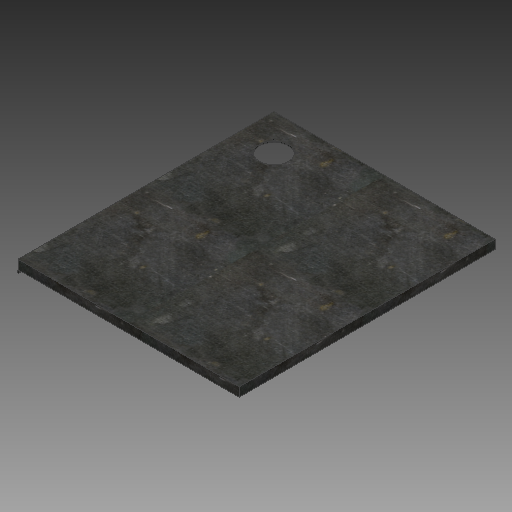
# Autodesk Inventor part: lid
Saved by Autodesk Inventor 2018 (Build 220112000, 112)
## iProperties
Created: 2018-08-03
Part Number: lid
Material: Steel
Document SubType Name: Modeling
Designer: Cole Tucker
Density: 7.85 g/cm^3
Appearance: Plate
Mass: 1610.8 g
Surface Area: 2598 cm^2
Volume: 205.197 cm^3
Author: Cole Tucker
Autodesk Inventor part; units mm, degrees
ref_plane "YZ Plane" through (0, 0, 0) normal (1, 0, 0) x (0, 1, 0)
ref_plane "XZ Plane" through (0, 0, 0) normal (0, 1, 0) x (-1, 0, 0)
ref_plane "XY Plane" through (0, 0, 0) normal (0, 0, 1) x (1, 0, 0)
sketch "Sketch1" plane through (0, 0, 0) normal (0, 1, 0) x (-1, 0, 0)
  line L0 (0, 0) -> (361.95, 0)
  line L1 (361.95, 0) -> (361.95, -312.7502)
  line L2 (361.95, -312.7502) -> (0, -312.7502)
  line L3 (0, -312.7502) -> (0, 0)
  dimension "d0" = 361.95
  dimension "d1" = 312.7502
  constraints: 8 end point, 2 parallel, 1 horizontal, 1 perpendicular
  measures "d0" distance of L1.end L2.end
  measures "d1" distance of L0.end L1.end
extrude "Extrusion1" add sketch "Sketch1" along normal blind 12.7
shell "Shell1" thickness 1.5875 removed faces 1 at (-120.65, 0, -104.2501)
sketch "Sketch2" plane through (0, 0, 0) normal (1, 0, 0) x (0, 0, -1)
  line L0 (0, 0) -> (0, -3.175)
  arc A0 (0, -1.5875) -> (1.5875, -3.175) centre (0, -3.175) ccw
  line L1 (1.5875, -3.175) -> (1.5875, 0)
  line L2 (312.7502, 0) -> (0, 0) projected
  line L3 (1.5875, 0) -> (0, 0)
  dimension "d5" = 3.175
  dimension "d6" = 3.175
  constraints: 6 end point, 2 point on circle, 2 vertical, 1 centre point, 1 coincident, 1 midpoint, 1 perpendicular, 1 tangent
  measures "d5" distance of L0.start L0.end
  measures "d6" diameter of A0
extrude "Extrusion2" add sketch "Sketch2" against normal up to surface (361.95 mm away)
sketch "Sketch3" plane through (0, 12.7, 0) normal (0, 1, 0) x (1, 0, 0)
  line L0 (-361.95, 312.7502) -> (-361.95, 0) construction
  line L1 (-361.95, 0) -> (-311.15, 0) construction
  line L2 (-311.15, 0) -> (-311.15, 50.8) construction
  line L3 (-311.15, 50.8) -> (-361.95, 50.8) construction
  line L4 (-361.95, 50.8) -> (-361.95, 0) construction
  circle A0 centre (-311.15, 50.8) radius 20.6375
  point P0 (0, 0)
  dimension "d9" = 50.8
  dimension "d10" = 50.8
  dimension "d11" = 41.275
  constraints: 8 end point, 2 parallel, 1 centre point, 1 coincident, 1 horizontal, 1 perpendicular
  measures "d9" distance of L3.end L2.end
  measures "d10" distance of L2.end L1.end
  measures "d11" diameter of A0
extrude "Extrusion3" cut sketch "Sketch3" against normal blind 12.7
sketch "Sketch4" plane through (0, 12.7, 0) normal (0, 1, 0) x (1, 0, 0)
  circle A0 centre (-311.15, 50.8) radius 20.6375 construction
  line L0 (-311.15, 50.8) -> (-295.0845, 50.8) construction
  line L1 (-295.0845, 50.8) -> (-295.0845, 66.8655) construction
  line L2 (-295.0845, 66.8655) -> (-311.15, 66.8655) construction
  line L3 (-311.15, 66.8655) -> (-311.15, 50.8) construction
  line L4 (-311.15, 50.8) -> (-327.2155, 50.8) construction
  line L5 (-327.2155, 50.8) -> (-327.2155, 34.7345) construction
  line L6 (-327.2155, 34.7345) -> (-311.15, 34.7345) construction
  line L7 (-311.15, 34.7345) -> (-311.15, 50.8) construction
  line L8 (-295.0845, 66.8655) -> (-327.2155, 66.8655)
  line L9 (-327.2155, 66.8655) -> (-327.2155, 34.7345)
  line L10 (-327.2155, 34.7345) -> (-295.0845, 34.7345)
  line L11 (-295.0845, 34.7345) -> (-295.0845, 66.8655)
  point P0 (0, 0)
  dimension "d14" = 16.0655
  dimension "d15" = 16.0655
  dimension "d16" = 16.0655
  dimension "d17" = 16.0655
  constraints: 24 end point, 6 parallel, 4 coincident, 3 horizontal, 3 perpendicular
  measures "d14" distance of L2.end L1.end
  measures "d15" distance of L1.end L0.end
  measures "d16" distance of L6.end L5.end
  measures "d17" distance of L5.end L4.end
hole "Hole1" at (-327.2155, 12.7, -66.8655) at (-295.0845, 12.7, -66.8655) at (-295.0845, 12.7, -34.7345) at (-327.2155, 12.7, -34.7345) direction (0, -1, 0) diameter 3.175 depth 25.4 tip angle 118
equation "\"d15\" = d14"
equation "\"d16\" = d14"
equation "\"d17\" = d14"
body "Solid1"
